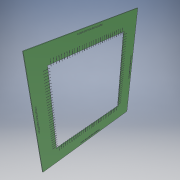
# Autodesk Inventor part: PCB-FerriteCore#01
Saved by Autodesk Inventor 2018 (Build 220112000, 112)
## iProperties
Created: 2025-02-18
Part Number: PCB-FerriteCore#01
Material: Železo, lité
Document SubType Name: Modeling
Designer: Jozko Mrkvicka
Density: 7.15 g/cm^3
Appearance: Železo – šedé
Author: Jozko Mrkvicka
Autodesk Inventor part; units mm, degrees
(part 1 of 3)
ref_plane "YZ Plane" through (0, 0, 0) normal (1, 0, 0) x (0, 1, 0)
ref_plane "XZ Plane" through (0, 0, 0) normal (0, 1, 0) x (-1, 0, 0)
ref_plane "XY Plane" through (0, 0, 0) normal (0, 0, 1) x (1, 0, 0)
sketch "Náčrt1" plane through (0, 0, 0) normal (0, 1, 0) x (-1, 0, 0)
  line L0 (-177.8, 177.8) -> (177.8, 177.8)
  line L1 (177.8, 177.8) -> (177.8, -177.8)
  line L2 (177.8, -177.8) -> (-177.8, -177.8)
  line L3 (-177.8, -177.8) -> (-177.8, 177.8)
  line L4 (-177.8, 177.8) -> (177.8, -177.8) construction
  line L5 (177.8, 177.8) -> (-177.8, -177.8) construction
  line L6 (-127, 127) -> (127, 127)
  line L7 (127, 127) -> (127, -127)
  line L8 (127, -127) -> (-127, -127)
  line L9 (-127, -127) -> (-127, 127)
  line L10 (-127, 127) -> (127, -127) construction
  line L11 (127, 127) -> (-127, -127) construction
  point P0 (0, 0)
  dimension "d2" = 355.6
  dimension "d3" = 355.6
  dimension "d4" = 254
  dimension "d5" = 254
  constraints: 24 end point, 4 midpoint, 4 parallel, 2 horizontal, 2 perpendicular
  measures "d2" distance of L1.end L2.end
  measures "d3" distance of L0.end L1.end
  measures "d4" distance of L7.end L8.end
  measures "d5" distance of L6.end L7.end
extrude "Vysunutí1" add sketch "Náčrt1" along normal blind 2.54
sketch "Náčrt2" plane through (0, 2.54, 0) normal (0, 1, 0) x (1, 0, 0)
  line L0 (88.9, -88.9) -> (-88.9, -88.9)
  line L1 (3.71, -139.7) -> (3.91, -139.7)
  line L2 (3.91, -139.7) -> (3.91, -121.92)
  line L3 (3.91, -121.92) -> (3.71, -121.92)
  line L4 (3.71, -121.92) -> (3.71, -139.7)
  line L5 (3.71, -139.7) -> (3.91, -121.92) construction
  line L6 (3.91, -139.7) -> (3.71, -121.92) construction
  line L7 (-248.92, 0) -> (248.92, 0) projected
  line L8 (0, 248.92) -> (0, -248.92) projected
  line L9 (3.71, 139.7) -> (3.91, 139.7)
  line L10 (3.91, 139.7) -> (3.91, 121.92)
  line L11 (3.91, 121.92) -> (3.71, 121.92)
  line L12 (3.71, 121.92) -> (3.71, 139.7)
  point P0 (0, 0)
  point P1 (3.81, -130.81)
  dimension "d18" = 3.81
  dimension "d19" = 0.2
  dimension "d20" = 17.78
  dimension "d24" = 139.7
  constraints: 22 end point, 4 symmetric about line, 3 parallel, 2 midpoint, 1 perpendicular
  measures "d18" horizontal distance of point (0, 0) point (3.81, -130.81)
  measures "d19" distance of L2.end L3.end
  measures "d20" distance of L1.end L2.end
  measures "d24" distance from line of L1 point (0, 0)
extrude "Vysunutí2" add sketch "Náčrt2" along normal blind 0.2
pattern_linear "Obdélníkové pole2" count 32 spacing 7.62 along (-1, 0, 0) of "Vysunutí2" first direction both ways yes
sketch "Náčrt3" plane through (0, 2.54, 0) normal (0, 1, 0) x (1, 0, 0)
  line L0 (-248.92, 0) -> (248.92, 0) projected
  line L1 (0, 248.92) -> (0, -248.92) projected
  line L2 (-121.92, -3.71) -> (-139.7, -3.71)
  line L3 (-139.7, -3.71) -> (-139.7, -3.91)
  line L4 (-139.7, -3.91) -> (-121.92, -3.91)
  line L5 (-121.92, -3.91) -> (-121.92, -3.71)
  line L6 (-121.92, -3.71) -> (-139.7, -3.91) construction
  line L7 (-139.7, -3.71) -> (-121.92, -3.91) construction
  line L8 (121.92, -3.71) -> (139.7, -3.71)
  line L9 (139.7, -3.71) -> (139.7, -3.91)
  line L10 (139.7, -3.91) -> (121.92, -3.91)
  line L11 (121.92, -3.91) -> (121.92, -3.71)
  point P0 (0, 0)
  point P1 (-130.81, -3.81)
  dimension "d35" = 0.2
  dimension "d36" = 17.78
  dimension "d37" = 3.81
  dimension "d38" = 139.7
  constraints: 20 end point, 4 symmetric about line, 2 midpoint, 2 parallel, 1 horizontal, 1 perpendicular
  measures "d35" distance of L4.end L2.start
  measures "d36" distance of L3.end L4.end
  measures "d37" distance from line of L0 point (-130.81, -3.81)
  measures "d38" distance between parallel lines of L1 L3
extrude "Vysunutí3" add sketch "Náčrt3" along normal blind 0.2
pattern_linear "Obdélníkové pole3" count 32 spacing 7.62 along (0, 0, -1) of "Vysunutí3" first direction both ways yes
sketch "Náčrt5" plane through (0, 2.54, 0) normal (0, 1, 0) x (1, 0, 0)
  line L0 (-248.92, 0) -> (248.92, 0) projected
  line L1 (172.72, -40.64) -> (167.64, -40.64)
  line L2 (167.64, -40.64) -> (167.64, 40.64)
  line L3 (167.64, 40.64) -> (172.72, 40.64)
  line L4 (172.72, 40.64) -> (172.72, -40.64)
  line L5 (172.72, -40.64) -> (167.64, 40.64) construction
  line L6 (167.64, -40.64) -> (172.72, 40.64) construction
  line L7 (177.8, -177.8) -> (177.8, 177.8) projected
  line L8 (177.8, 177.8) -> (-177.8, 177.8) projected
  line L9 (-177.8, 177.8) -> (-177.8, -177.8) projected
  line L10 (169.2275, 39.6875) -> (168.5925, 39.6875)
  line L11 (168.5925, 39.6875) -> (168.5925, 39.0525)
  line L12 (168.5925, 39.0525) -> (169.2275, 39.0525)
  line L13 (169.2275, 39.0525) -> (169.2275, 39.6875)
  line L14 (169.2275, 39.6875) -> (168.5925, 39.0525) construction
  line L15 (168.5925, 39.6875) -> (169.2275, 39.0525) construction
  line L16 (0, 248.92) -> (0, -248.92) projected
  line L17 (40.64, -167.64) -> (-40.64, -167.64)
  line L18 (-40.64, -167.64) -> (-40.64, -172.72)
  line L19 (-40.64, -172.72) -> (40.64, -172.72)
  line L20 (40.64, -172.72) -> (40.64, -167.64)
  line L21 (40.64, -167.64) -> (-40.64, -172.72) construction
  line L22 (-40.64, -167.64) -> (40.64, -172.72) construction
  line L23 (-177.8, -177.8) -> (177.8, -177.8) projected
  line L24 (40.64, 172.72) -> (-40.64, 172.72)
  line L25 (-40.64, 172.72) -> (-40.64, 167.64)
  line L26 (-40.64, 167.64) -> (40.64, 167.64)
  line L27 (40.64, 167.64) -> (40.64, 172.72)
  line L28 (40.64, 172.72) -> (-40.64, 167.64) construction
  line L29 (-40.64, 172.72) -> (40.64, 167.64) construction
  line L30 (-39.0525, -171.1325) -> (-39.6875, -171.1325)
  line L31 (-39.6875, -171.1325) -> (-39.6875, -171.7675)
  line L32 (-39.6875, -171.7675) -> (-39.0525, -171.7675)
  line L33 (-39.0525, -171.7675) -> (-39.0525, -171.1325)
  line L34 (-39.0525, -171.1325) -> (-39.6875, -171.7675) construction
  line L35 (-39.6875, -171.1325) -> (-39.0525, -171.7675) construction
  line L36 (-36.5125, -171.1325) -> (-37.1475, -171.1325)
  line L37 (-36.5125, -171.7675) -> (-36.5125, -171.1325)
  line L38 (-37.1475, -171.1325) -> (-37.1475, -171.7675)
  line L39 (-37.1475, -171.7675) -> (-36.5125, -171.7675)
  line L40 (-36.5125, -171.1325) -> (-37.1475, -171.7675) construction
  line L41 (-37.1475, -171.1325) -> (-36.5125, -171.7675) construction
  line L42 (-33.9725, -171.1325) -> (-34.6075, -171.1325)
  line L43 (-33.9725, -171.7675) -> (-33.9725, -171.1325)
  line L44 (-34.6075, -171.1325) -> (-34.6075, -171.7675)
  line L45 (-34.6075, -171.7675) -> (-33.9725, -171.7675)
  line L46 (-33.9725, -171.1325) -> (-34.6075, -171.7675) construction
  line L47 (-34.6075, -171.1325) -> (-33.9725, -171.7675) construction
  line L48 (-31.4325, -171.1325) -> (-32.0675, -171.1325)
  line L49 (-31.4325, -171.7675) -> (-31.4325, -171.1325)
  line L50 (-32.0675, -171.1325) -> (-32.0675, -171.7675)
  line L51 (-32.0675, -171.7675) -> (-31.4325, -171.7675)
  line L52 (-31.4325, -171.1325) -> (-32.0675, -171.7675) construction
  line L53 (-32.0675, -171.1325) -> (-31.4325, -171.7675) construction
  line L54 (-28.8925, -171.1325) -> (-29.5275, -171.1325)
  line L55 (-28.8925, -171.7675) -> (-28.8925, -171.1325)
  line L56 (-29.5275, -171.1325) -> (-29.5275, -171.7675)
  line L57 (-29.5275, -171.7675) -> (-28.8925, -171.7675)
  line L58 (-28.8925, -171.1325) -> (-29.5275, -171.7675) construction
  line L59 (-29.5275, -171.1325) -> (-28.8925, -171.7675) construction
  line L60 (-26.3525, -171.1325) -> (-26.9875, -171.1325)
  line L61 (-26.3525, -171.7675) -> (-26.3525, -171.1325)
  line L62 (-26.9875, -171.1325) -> (-26.9875, -171.7675)
  line L63 (-26.9875, -171.7675) -> (-26.3525, -171.7675)
  line L64 (-26.3525, -171.1325) -> (-26.9875, -171.7675) construction
  line L65 (-26.9875, -171.1325) -> (-26.3525, -171.7675) construction
  line L66 (-23.8125, -171.1325) -> (-24.4475, -171.1325)
  line L67 (-23.8125, -171.7675) -> (-23.8125, -171.1325)
  line L68 (-24.4475, -171.1325) -> (-24.4475, -171.7675)
  line L69 (-24.4475, -171.7675) -> (-23.8125, -171.7675)
  line L70 (-23.8125, -171.1325) -> (-24.4475, -171.7675) construction
  line L71 (-24.4475, -171.1325) -> (-23.8125, -171.7675) construction
  line L72 (-21.2725, -171.1325) -> (-21.9075, -171.1325)
  line L73 (-21.2725, -171.7675) -> (-21.2725, -171.1325)
  line L74 (-21.9075, -171.1325) -> (-21.9075, -171.7675)
  line L75 (-21.9075, -171.7675) -> (-21.2725, -171.7675)
  line L76 (-21.2725, -171.1325) -> (-21.9075, -171.7675) construction
  line L77 (-21.9075, -171.1325) -> (-21.2725, -171.7675) construction
  line L78 (-18.7325, -171.1325) -> (-19.3675, -171.1325)
  line L79 (-18.7325, -171.7675) -> (-18.7325, -171.1325)
  line L80 (-19.3675, -171.1325) -> (-19.3675, -171.7675)
  line L81 (-19.3675, -171.7675) -> (-18.7325, -171.7675)
  line L82 (-18.7325, -171.1325) -> (-19.3675, -171.7675) construction
  line L83 (-19.3675, -171.1325) -> (-18.7325, -171.7675) construction
  line L84 (-16.1925, -171.1325) -> (-16.8275, -171.1325)
  line L85 (-16.1925, -171.7675) -> (-16.1925, -171.1325)
  line L86 (-16.8275, -171.1325) -> (-16.8275, -171.7675)
  line L87 (-16.8275, -171.7675) -> (-16.1925, -171.7675)
  line L88 (-16.1925, -171.1325) -> (-16.8275, -171.7675) construction
  line L89 (-16.8275, -171.1325) -> (-16.1925, -171.7675) construction
  line L90 (-13.6525, -171.1325) -> (-14.2875, -171.1325)
  line L91 (-13.6525, -171.7675) -> (-13.6525, -171.1325)
  line L92 (-14.2875, -171.1325) -> (-14.2875, -171.7675)
  line L93 (-14.2875, -171.7675) -> (-13.6525, -171.7675)
  line L94 (-13.6525, -171.1325) -> (-14.2875, -171.7675) construction
  line L95 (-14.2875, -171.1325) -> (-13.6525, -171.7675) construction
  line L96 (-11.1125, -171.1325) -> (-11.7475, -171.1325)
  line L97 (-11.1125, -171.7675) -> (-11.1125, -171.1325)
  line L98 (-11.7475, -171.1325) -> (-11.7475, -171.7675)
  line L99 (-11.7475, -171.7675) -> (-11.1125, -171.7675)
  line L100 (-11.1125, -171.1325) -> (-11.7475, -171.7675) construction
  line L101 (-11.7475, -171.1325) -> (-11.1125, -171.7675) construction
  line L102 (-8.5725, -171.1325) -> (-9.2075, -171.1325)
  line L103 (-8.5725, -171.7675) -> (-8.5725, -171.1325)
  line L104 (-9.2075, -171.1325) -> (-9.2075, -171.7675)
  line L105 (-9.2075, -171.7675) -> (-8.5725, -171.7675)
  line L106 (-8.5725, -171.1325) -> (-9.2075, -171.7675) construction
  line L107 (-9.2075, -171.1325) -> (-8.5725, -171.7675) construction
  line L108 (-6.0325, -171.1325) -> (-6.6675, -171.1325)
  line L109 (-6.0325, -171.7675) -> (-6.0325, -171.1325)
  line L110 (-6.6675, -171.1325) -> (-6.6675, -171.7675)
  line L111 (-6.6675, -171.7675) -> (-6.0325, -171.7675)
  line L112 (-6.0325, -171.1325) -> (-6.6675, -171.7675) construction
  line L113 (-6.6675, -171.1325) -> (-6.0325, -171.7675) construction
  line L114 (-3.4925, -171.1325) -> (-4.1275, -171.1325)
  line L115 (-3.4925, -171.7675) -> (-3.4925, -171.1325)
  line L116 (-4.1275, -171.1325) -> (-4.1275, -171.7675)
  line L117 (-4.1275, -171.7675) -> (-3.4925, -171.7675)
  line L118 (-3.4925, -171.1325) -> (-4.1275, -171.7675) construction
  line L119 (-4.1275, -171.1325) -> (-3.4925, -171.7675) construction
  line L120 (-0.9525, -171.1325) -> (-1.5875, -171.1325)
  line L121 (-0.9525, -171.7675) -> (-0.9525, -171.1325)
  line L122 (-1.5875, -171.1325) -> (-1.5875, -171.7675)
  line L123 (-1.5875, -171.7675) -> (-0.9525, -171.7675)
  line L124 (-0.9525, -171.1325) -> (-1.5875, -171.7675) construction
  line L125 (-1.5875, -171.1325) -> (-0.9525, -171.7675) construction
  line L126 (1.5875, -171.1325) -> (0.9525, -171.1325)
  line L127 (1.5875, -171.7675) -> (1.5875, -171.1325)
  line L128 (0.9525, -171.1325) -> (0.9525, -171.7675)
  line L129 (0.9525, -171.7675) -> (1.5875, -171.7675)
  line L130 (1.5875, -171.1325) -> (0.9525, -171.7675) construction
  line L131 (0.9525, -171.1325) -> (1.5875, -171.7675) construction
  line L132 (4.1275, -171.1325) -> (3.4925, -171.1325)
  line L133 (4.1275, -171.7675) -> (4.1275, -171.1325)
  line L134 (3.4925, -171.1325) -> (3.4925, -171.7675)
  line L135 (3.4925, -171.7675) -> (4.1275, -171.7675)
  line L136 (4.1275, -171.1325) -> (3.4925, -171.7675) construction
  line L137 (3.4925, -171.1325) -> (4.1275, -171.7675) construction
  line L138 (6.6675, -171.1325) -> (6.0325, -171.1325)
  line L139 (6.6675, -171.7675) -> (6.6675, -171.1325)
  line L140 (6.0325, -171.1325) -> (6.0325, -171.7675)
  line L141 (6.0325, -171.7675) -> (6.6675, -171.7675)
  line L142 (6.6675, -171.1325) -> (6.0325, -171.7675) construction
  line L143 (6.0325, -171.1325) -> (6.6675, -171.7675) construction
  line L144 (9.2075, -171.1325) -> (8.5725, -171.1325)
  line L145 (9.2075, -171.7675) -> (9.2075, -171.1325)
  line L146 (8.5725, -171.1325) -> (8.5725, -171.7675)
  line L147 (8.5725, -171.7675) -> (9.2075, -171.7675)
  line L148 (9.2075, -171.1325) -> (8.5725, -171.7675) construction
  line L149 (8.5725, -171.1325) -> (9.2075, -171.7675) construction
  line L150 (11.7475, -171.1325) -> (11.1125, -171.1325)
  line L151 (11.7475, -171.7675) -> (11.7475, -171.1325)
  line L152 (11.1125, -171.1325) -> (11.1125, -171.7675)
  line L153 (11.1125, -171.7675) -> (11.7475, -171.7675)
  line L154 (11.7475, -171.1325) -> (11.1125, -171.7675) construction
  line L155 (11.1125, -171.1325) -> (11.7475, -171.7675) construction
  line L156 (14.2875, -171.1325) -> (13.6525, -171.1325)
  line L157 (14.2875, -171.7675) -> (14.2875, -171.1325)
  line L158 (13.6525, -171.1325) -> (13.6525, -171.7675)
  line L159 (13.6525, -171.7675) -> (14.2875, -171.7675)
  line L160 (14.2875, -171.1325) -> (13.6525, -171.7675) construction
  line L161 (13.6525, -171.1325) -> (14.2875, -171.7675) construction
  line L162 (16.8275, -171.1325) -> (16.1925, -171.1325)
  line L163 (16.8275, -171.7675) -> (16.8275, -171.1325)
  line L164 (16.1925, -171.1325) -> (16.1925, -171.7675)
  line L165 (16.1925, -171.7675) -> (16.8275, -171.7675)
  line L166 (16.8275, -171.1325) -> (16.1925, -171.7675) construction
  line L167 (16.1925, -171.1325) -> (16.8275, -171.7675) construction
  line L168 (19.3675, -171.1325) -> (18.7325, -171.1325)
  line L169 (19.3675, -171.7675) -> (19.3675, -171.1325)
  line L170 (18.7325, -171.1325) -> (18.7325, -171.7675)
  line L171 (18.7325, -171.7675) -> (19.3675, -171.7675)
  line L172 (19.3675, -171.1325) -> (18.7325, -171.7675) construction
  line L173 (18.7325, -171.1325) -> (19.3675, -171.7675) construction
  line L174 (21.9075, -171.1325) -> (21.2725, -171.1325)
  line L175 (21.9075, -171.7675) -> (21.9075, -171.1325)
  line L176 (21.2725, -171.1325) -> (21.2725, -171.7675)
  line L177 (21.2725, -171.7675) -> (21.9075, -171.7675)
  line L178 (21.9075, -171.1325) -> (21.2725, -171.7675) construction
  line L179 (21.2725, -171.1325) -> (21.9075, -171.7675) construction
  line L180 (24.4475, -171.1325) -> (23.8125, -171.1325)
  line L181 (24.4475, -171.7675) -> (24.4475, -171.1325)
  line L182 (23.8125, -171.1325) -> (23.8125, -171.7675)
  line L183 (23.8125, -171.7675) -> (24.4475, -171.7675)
  line L184 (24.4475, -171.1325) -> (23.8125, -171.7675) construction
  line L185 (23.8125, -171.1325) -> (24.4475, -171.7675) construction
  line L186 (26.9875, -171.1325) -> (26.3525, -171.1325)
  line L187 (26.9875, -171.7675) -> (26.9875, -171.1325)
  line L188 (26.3525, -171.1325) -> (26.3525, -171.7675)
  line L189 (26.3525, -171.7675) -> (26.9875, -171.7675)
  line L190 (26.9875, -171.1325) -> (26.3525, -171.7675) construction
  line L191 (26.3525, -171.1325) -> (26.9875, -171.7675) construction
  line L192 (29.5275, -171.1325) -> (28.8925, -171.1325)
  line L193 (29.5275, -171.7675) -> (29.5275, -171.1325)
  line L194 (28.8925, -171.1325) -> (28.8925, -171.7675)
  line L195 (28.8925, -171.7675) -> (29.5275, -171.7675)
  line L196 (29.5275, -171.1325) -> (28.8925, -171.7675) construction
  line L197 (28.8925, -171.1325) -> (29.5275, -171.7675) construction
  line L198 (32.0675, -171.1325) -> (31.4325, -171.1325)
  line L199 (32.0675, -171.7675) -> (32.0675, -171.1325)
  line L200 (31.4325, -171.1325) -> (31.4325, -171.7675)
  line L201 (31.4325, -171.7675) -> (32.0675, -171.7675)
  line L202 (32.0675, -171.1325) -> (31.4325, -171.7675) construction
  line L203 (31.4325, -171.1325) -> (32.0675, -171.7675) construction
  line L204 (34.6075, -171.1325) -> (33.9725, -171.1325)
  line L205 (34.6075, -171.7675) -> (34.6075, -171.1325)
  line L206 (33.9725, -171.1325) -> (33.9725, -171.7675)
  line L207 (33.9725, -171.7675) -> (34.6075, -171.7675)
  line L208 (34.6075, -171.1325) -> (33.9725, -171.7675) construction
  line L209 (33.9725, -171.1325) -> (34.6075, -171.7675) construction
  line L210 (37.1475, -171.1325) -> (36.5125, -171.1325)
  line L211 (37.1475, -171.7675) -> (37.1475, -171.1325)
  line L212 (36.5125, -171.1325) -> (36.5125, -171.7675)
  line L213 (36.5125, -171.7675) -> (37.1475, -171.7675)
  line L214 (37.1475, -171.1325) -> (36.5125, -171.7675) construction
  line L215 (36.5125, -171.1325) -> (37.1475, -171.7675) construction
  line L216 (39.6875, -171.1325) -> (39.0525, -171.1325)
  line L217 (39.6875, -171.7675) -> (39.6875, -171.1325)
  line L218 (39.0525, -171.1325) -> (39.0525, -171.7675)
  line L219 (39.0525, -171.7675) -> (39.6875, -171.7675)
  line L220 (39.6875, -171.1325) -> (39.0525, -171.7675) construction
  line L221 (39.0525, -171.1325) -> (39.6875, -171.7675) construction
  line L222 (-39.0525, -168.5925) -> (-39.6875, -168.5925)
  line L223 (-39.0525, -169.2275) -> (-39.0525, -168.5925)
  line L224 (-39.6875, -168.5925) -> (-39.6875, -169.2275)
  line L225 (-39.6875, -169.2275) -> (-39.0525, -169.2275)
  line L226 (-39.0525, -168.5925) -> (-39.6875, -169.2275) construction
  line L227 (-39.6875, -168.5925) -> (-39.0525, -169.2275) construction
  line L228 (-36.5125, -168.5925) -> (-37.1475, -168.5925)
  line L229 (-36.5125, -169.2275) -> (-36.5125, -168.5925)
  line L230 (-37.1475, -168.5925) -> (-37.1475, -169.2275)
  line L231 (-37.1475, -169.2275) -> (-36.5125, -169.2275)
  line L232 (-36.5125, -168.5925) -> (-37.1475, -169.2275) construction
  line L233 (-37.1475, -168.5925) -> (-36.5125, -169.2275) construction
  line L234 (-33.9725, -168.5925) -> (-34.6075, -168.5925)
  line L235 (-33.9725, -169.2275) -> (-33.9725, -168.5925)
  line L236 (-34.6075, -168.5925) -> (-34.6075, -169.2275)
  line L237 (-34.6075, -169.2275) -> (-33.9725, -169.2275)
  line L238 (-33.9725, -168.5925) -> (-34.6075, -169.2275) construction
  line L239 (-34.6075, -168.5925) -> (-33.9725, -169.2275) construction
  line L240 (-31.4325, -168.5925) -> (-32.0675, -168.5925)
  line L241 (-31.4325, -169.2275) -> (-31.4325, -168.5925)
  line L242 (-32.0675, -168.5925) -> (-32.0675, -169.2275)
  line L243 (-32.0675, -169.2275) -> (-31.4325, -169.2275)
  line L244 (-31.4325, -168.5925) -> (-32.0675, -169.2275) construction
  line L245 (-32.0675, -168.5925) -> (-31.4325, -169.2275) construction
  line L246 (-28.8925, -168.5925) -> (-29.5275, -168.5925)
  line L247 (-28.8925, -169.2275) -> (-28.8925, -168.5925)
  line L248 (-29.5275, -168.5925) -> (-29.5275, -169.2275)
  line L249 (-29.5275, -169.2275) -> (-28.8925, -169.2275)
  line L250 (-28.8925, -168.5925) -> (-29.5275, -169.2275) construction
  line L251 (-29.5275, -168.5925) -> (-28.8925, -169.2275) construction
  line L252 (-26.3525, -168.5925) -> (-26.9875, -168.5925)
  line L253 (-26.3525, -169.2275) -> (-26.3525, -168.5925)
  line L254 (-26.9875, -168.5925) -> (-26.9875, -169.2275)
  line L255 (-26.9875, -169.2275) -> (-26.3525, -169.2275)
  line L256 (-26.3525, -168.5925) -> (-26.9875, -169.2275) construction
  line L257 (-26.9875, -168.5925) -> (-26.3525, -169.2275) construction
  line L258 (-23.8125, -168.5925) -> (-24.4475, -168.5925)
  line L259 (-23.8125, -169.2275) -> (-23.8125, -168.5925)
  line L260 (-24.4475, -168.5925) -> (-24.4475, -169.2275)
  line L261 (-24.4475, -169.2275) -> (-23.8125, -169.2275)
  line L262 (-23.8125, -168.5925) -> (-24.4475, -169.2275) construction
  line L263 (-24.4475, -168.5925) -> (-23.8125, -169.2275) construction
  line L264 (-21.2725, -168.5925) -> (-21.9075, -168.5925)
  line L265 (-21.2725, -169.2275) -> (-21.2725, -168.5925)
  line L266 (-21.9075, -168.5925) -> (-21.9075, -169.2275)
  line L267 (-21.9075, -169.2275) -> (-21.2725, -169.2275)
  line L268 (-21.2725, -168.5925) -> (-21.9075, -169.2275) construction
  line L269 (-21.9075, -168.5925) -> (-21.2725, -169.2275) construction
  line L270 (-18.7325, -168.5925) -> (-19.3675, -168.5925)
  line L271 (-18.7325, -169.2275) -> (-18.7325, -168.5925)
  line L272 (-19.3675, -168.5925) -> (-19.3675, -169.2275)
  line L273 (-19.3675, -169.2275) -> (-18.7325, -169.2275)
  line L274 (-18.7325, -168.5925) -> (-19.3675, -169.2275) construction
  line L275 (-19.3675, -168.5925) -> (-18.7325, -169.2275) construction
  line L276 (-16.1925, -168.5925) -> (-16.8275, -168.5925)
  line L277 (-16.1925, -169.2275) -> (-16.1925, -168.5925)
  line L278 (-16.8275, -168.5925) -> (-16.8275, -169.2275)
  line L279 (-16.8275, -169.2275) -> (-16.1925, -169.2275)
  line L280 (-16.1925, -168.5925) -> (-16.8275, -169.2275) construction
  line L281 (-16.8275, -168.5925) -> (-16.1925, -169.2275) construction
  line L282 (-13.6525, -168.5925) -> (-14.2875, -168.5925)
  line L283 (-13.6525, -169.2275) -> (-13.6525, -168.5925)
  line L284 (-14.2875, -168.5925) -> (-14.2875, -169.2275)
  line L285 (-14.2875, -169.2275) -> (-13.6525, -169.2275)
  line L286 (-13.6525, -168.5925) -> (-14.2875, -169.2275) construction
  line L287 (-14.2875, -168.5925) -> (-13.6525, -169.2275) construction
  line L288 (-11.1125, -168.5925) -> (-11.7475, -168.5925)
  line L289 (-11.1125, -169.2275) -> (-11.1125, -168.5925)
  line L290 (-11.7475, -168.5925) -> (-11.7475, -169.2275)
  line L291 (-11.7475, -169.2275) -> (-11.1125, -169.2275)
  line L292 (-11.1125, -168.5925) -> (-11.7475, -169.2275) construction
  line L293 (-11.7475, -168.5925) -> (-11.1125, -169.2275) construction
  line L294 (-8.5725, -168.5925) -> (-9.2075, -168.5925)
  line L295 (-8.5725, -169.2275) -> (-8.5725, -168.5925)
  line L296 (-9.2075, -168.5925) -> (-9.2075, -169.2275)
  line L297 (-9.2075, -169.2275) -> (-8.5725, -169.2275)
  line L298 (-8.5725, -168.5925) -> (-9.2075, -169.2275) construction
  line L299 (-9.2075, -168.5925) -> (-8.5725, -169.2275) construction
  line L300 (-6.0325, -168.5925) -> (-6.6675, -168.5925)
  line L301 (-6.0325, -169.2275) -> (-6.0325, -168.5925)
  line L302 (-6.6675, -168.5925) -> (-6.6675, -169.2275)
  line L303 (-6.6675, -169.2275) -> (-6.0325, -169.2275)
  line L304 (-6.0325, -168.5925) -> (-6.6675, -169.2275) construction
  line L305 (-6.6675, -168.5925) -> (-6.0325, -169.2275) construction
  line L306 (-3.4925, -168.5925) -> (-4.1275, -168.5925)
  line L307 (-3.4925, -169.2275) -> (-3.4925, -168.5925)
  line L308 (-4.1275, -168.5925) -> (-4.1275, -169.2275)
  line L309 (-4.1275, -169.2275) -> (-3.4925, -169.2275)
  line L310 (-3.4925, -168.5925) -> (-4.1275, -169.2275) construction
  line L311 (-4.1275, -168.5925) -> (-3.4925, -169.2275) construction
  line L312 (-0.9525, -168.5925) -> (-1.5875, -168.5925)
  line L313 (-0.9525, -169.2275) -> (-0.9525, -168.5925)
  line L314 (-1.5875, -168.5925) -> (-1.5875, -169.2275)
  line L315 (-1.5875, -169.2275) -> (-0.9525, -169.2275)
  line L316 (-0.9525, -168.5925) -> (-1.5875, -169.2275) construction
  line L317 (-1.5875, -168.5925) -> (-0.9525, -169.2275) construction
  line L318 (1.5875, -168.5925) -> (0.9525, -168.5925)
  line L319 (1.5875, -169.2275) -> (1.5875, -168.5925)
  line L320 (0.9525, -168.5925) -> (0.9525, -169.2275)
  line L321 (0.9525, -169.2275) -> (1.5875, -169.2275)
  line L322 (1.5875, -168.5925) -> (0.9525, -169.2275) construction
  line L323 (0.9525, -168.5925) -> (1.5875, -169.2275) construction
  line L324 (4.1275, -168.5925) -> (3.4925, -168.5925)
  line L325 (4.1275, -169.2275) -> (4.1275, -168.5925)
  line L326 (3.4925, -168.5925) -> (3.4925, -169.2275)
  line L327 (3.4925, -169.2275) -> (4.1275, -169.2275)
  line L328 (4.1275, -168.5925) -> (3.4925, -169.2275) construction
  line L329 (3.4925, -168.5925) -> (4.1275, -169.2275) construction
  line L330 (6.6675, -168.5925) -> (6.0325, -168.5925)
  line L331 (6.6675, -169.2275) -> (6.6675, -168.5925)
  line L332 (6.0325, -168.5925) -> (6.0325, -169.2275)
  line L333 (6.0325, -169.2275) -> (6.6675, -169.2275)
  line L334 (6.6675, -168.5925) -> (6.0325, -169.2275) construction
  line L335 (6.0325, -168.5925) -> (6.6675, -169.2275) construction
  line L336 (9.2075, -168.5925) -> (8.5725, -168.5925)
  line L337 (9.2075, -169.2275) -> (9.2075, -168.5925)
  line L338 (8.5725, -168.5925) -> (8.5725, -169.2275)
  line L339 (8.5725, -169.2275) -> (9.2075, -169.2275)
  line L340 (9.2075, -168.5925) -> (8.5725, -169.2275) construction
  line L341 (8.5725, -168.5925) -> (9.2075, -169.2275) construction
  line L342 (11.7475, -168.5925) -> (11.1125, -168.5925)
  line L343 (11.7475, -169.2275) -> (11.7475, -168.5925)
  line L344 (11.1125, -168.5925) -> (11.1125, -169.2275)
  line L345 (11.1125, -169.2275) -> (11.7475, -169.2275)
  line L346 (11.7475, -168.5925) -> (11.1125, -169.2275) construction
  line L347 (11.1125, -168.5925) -> (11.7475, -169.2275) construction
  line L348 (14.2875, -168.5925) -> (13.6525, -168.5925)
  line L349 (14.2875, -169.2275) -> (14.2875, -168.5925)
  line L350 (13.6525, -168.5925) -> (13.6525, -169.2275)
  line L351 (13.6525, -169.2275) -> (14.2875, -169.2275)
  line L352 (14.2875, -168.5925) -> (13.6525, -169.2275) construction
  line L353 (13.6525, -168.5925) -> (14.2875, -169.2275) construction
  line L354 (16.8275, -168.5925) -> (16.1925, -168.5925)
  line L355 (16.8275, -169.2275) -> (16.8275, -168.5925)
  line L356 (16.1925, -168.5925) -> (16.1925, -169.2275)
  line L357 (16.1925, -169.2275) -> (16.8275, -169.2275)
  line L358 (16.8275, -168.5925) -> (16.1925, -169.2275) construction
  line L359 (16.1925, -168.5925) -> (16.8275, -169.2275) construction
  line L360 (19.3675, -168.5925) -> (18.7325, -168.5925)
  line L361 (19.3675, -169.2275) -> (19.3675, -168.5925)
  line L362 (18.7325, -168.5925) -> (18.7325, -169.2275)
  line L363 (18.7325, -169.2275) -> (19.3675, -169.2275)
  line L364 (19.3675, -168.5925) -> (18.7325, -169.2275) construction
  line L365 (18.7325, -168.5925) -> (19.3675, -169.2275) construction
  line L366 (21.9075, -168.5925) -> (21.2725, -168.5925)
  line L367 (21.9075, -169.2275) -> (21.9075, -168.5925)
  line L368 (21.2725, -168.5925) -> (21.2725, -169.2275)
  line L369 (21.2725, -169.2275) -> (21.9075, -169.2275)
  line L370 (21.9075, -168.5925) -> (21.2725, -169.2275) construction
  line L371 (21.2725, -168.5925) -> (21.9075, -169.2275) construction
  line L372 (24.4475, -168.5925) -> (23.8125, -168.5925)
  line L373 (24.4475, -169.2275) -> (24.4475, -168.5925)
  line L374 (23.8125, -168.5925) -> (23.8125, -169.2275)
  line L375 (23.8125, -169.2275) -> (24.4475, -169.2275)
  line L376 (24.4475, -168.5925) -> (23.8125, -169.2275) construction
  line L377 (23.8125, -168.5925) -> (24.4475, -169.2275) construction
  line L378 (26.9875, -168.5925) -> (26.3525, -168.5925)
  line L379 (26.9875, -169.2275) -> (26.9875, -168.5925)
  line L380 (26.3525, -168.5925) -> (26.3525, -169.2275)
  line L381 (26.3525, -169.2275) -> (26.9875, -169.2275)
  line L382 (26.9875, -168.5925) -> (26.3525, -169.2275) construction
  line L383 (26.3525, -168.5925) -> (26.9875, -169.2275) construction
  line L384 (29.5275, -168.5925) -> (28.8925, -168.5925)
  line L385 (29.5275, -169.2275) -> (29.5275, -168.5925)
  line L386 (28.8925, -168.5925) -> (28.8925, -169.2275)
  line L387 (28.8925, -169.2275) -> (29.5275, -169.2275)
  line L388 (29.5275, -168.5925) -> (28.8925, -169.2275) construction
  line L389 (28.8925, -168.5925) -> (29.5275, -169.2275) construction
  line L390 (32.0675, -168.5925) -> (31.4325, -168.5925)
  line L391 (32.0675, -169.2275) -> (32.0675, -168.5925)
  line L392 (31.4325, -168.5925) -> (31.4325, -169.2275)
  line L393 (31.4325, -169.2275) -> (32.0675, -169.2275)
  line L394 (32.0675, -168.5925) -> (31.4325, -169.2275) construction
  line L395 (31.4325, -168.5925) -> (32.0675, -169.2275) construction
  line L396 (34.6075, -168.5925) -> (33.9725, -168.5925)
  line L397 (34.6075, -169.2275) -> (34.6075, -168.5925)
  line L398 (33.9725, -168.5925) -> (33.9725, -169.2275)
  line L399 (33.9725, -169.2275) -> (34.6075, -169.2275)
  line L400 (34.6075, -168.5925) -> (33.9725, -169.2275) construction
  line L401 (33.9725, -168.5925) -> (34.6075, -169.2275) construction
  line L402 (37.1475, -168.5925) -> (36.5125, -168.5925)
  line L403 (37.1475, -169.2275) -> (37.1475, -168.5925)
  line L404 (36.5125, -168.5925) -> (36.5125, -169.2275)
  line L405 (36.5125, -169.2275) -> (37.1475, -169.2275)
  line L406 (37.1475, -168.5925) -> (36.5125, -169.2275) construction
  line L407 (36.5125, -168.5925) -> (37.1475, -169.2275) construction
  line L408 (39.6875, -168.5925) -> (39.0525, -168.5925)
  line L409 (39.6875, -169.2275) -> (39.6875, -168.5925)
  line L410 (39.0525, -168.5925) -> (39.0525, -169.2275)
  line L411 (39.0525, -169.2275) -> (39.6875, -169.2275)
  line L412 (39.6875, -168.5925) -> (39.0525, -169.2275) construction
  line L413 (39.0525, -168.5925) -> (39.6875, -169.2275) construction
  line L414 (-39.0525, 169.2275) -> (-39.6875, 169.2275)
  line L415 (-39.6875, 169.2275) -> (-39.6875, 168.5925)
  line L416 (-39.6875, 168.5925) -> (-39.0525, 168.5925)
  line L417 (-39.0525, 168.5925) -> (-39.0525, 169.2275)
  line L418 (-39.0525, 169.2275) -> (-39.6875, 168.5925) construction
  line L419 (-39.6875, 169.2275) -> (-39.0525, 168.5925) construction
  line L420 (-37.1475, 168.5925) -> (-36.5125, 168.5925)
  line L421 (-36.5125, 168.5925) -> (-36.5125, 169.2275)
  line L422 (-37.1475, 169.2275) -> (-37.1475, 168.5925)
  line L423 (-36.5125, 169.2275) -> (-37.1475, 169.2275)
  line L424 (-36.5125, 169.2275) -> (-37.1475, 168.5925) construction
  line L425 (-37.1475, 169.2275) -> (-36.5125, 168.5925) construction
  line L426 (-34.6075, 168.5925) -> (-33.9725, 168.5925)
  line L427 (-33.9725, 168.5925) -> (-33.9725, 169.2275)
  line L428 (-34.6075, 169.2275) -> (-34.6075, 168.5925)
  line L429 (-33.9725, 169.2275) -> (-34.6075, 169.2275)
  line L430 (-33.9725, 169.2275) -> (-34.6075, 168.5925) construction
  line L431 (-34.6075, 169.2275) -> (-33.9725, 168.5925) construction
  line L432 (-32.0675, 168.5925) -> (-31.4325, 168.5925)
  line L433 (-31.4325, 168.5925) -> (-31.4325, 169.2275)
  line L434 (-32.0675, 169.2275) -> (-32.0675, 168.5925)
  line L435 (-31.4325, 169.2275) -> (-32.0675, 169.2275)
  line L436 (-31.4325, 169.2275) -> (-32.0675, 168.5925) construction
  line L437 (-32.0675, 169.2275) -> (-31.4325, 168.5925) construction
  line L438 (-29.5275, 168.5925) -> (-28.8925, 168.5925)
  line L439 (-28.8925, 168.5925) -> (-28.8925, 169.2275)
  line L440 (-29.5275, 169.2275) -> (-29.5275, 168.5925)
  line L441 (-28.8925, 169.2275) -> (-29.5275, 169.2275)
  line L442 (-28.8925, 169.2275) -> (-29.5275, 168.5925) construction
  line L443 (-29.5275, 169.2275) -> (-28.8925, 168.5925) construction
  line L444 (-26.9875, 168.5925) -> (-26.3525, 168.5925)
  line L445 (-26.3525, 168.5925) -> (-26.3525, 169.2275)
  line L446 (-26.9875, 169.2275) -> (-26.9875, 168.5925)
  line L447 (-26.3525, 169.2275) -> (-26.9875, 169.2275)
  line L448 (-26.3525, 169.2275) -> (-26.9875, 168.5925) construction
  line L449 (-26.9875, 169.2275) -> (-26.3525, 168.5925) construction
  line L450 (-24.4475, 168.5925) -> (-23.8125, 168.5925)
  line L451 (-23.8125, 168.5925) -> (-23.8125, 169.2275)
  line L452 (-24.4475, 169.2275) -> (-24.4475, 168.5925)
  line L453 (-23.8125, 169.2275) -> (-24.4475, 169.2275)
  line L454 (-23.8125, 169.2275) -> (-24.4475, 168.5925) construction
  line L455 (-24.4475, 169.2275) -> (-23.8125, 168.5925) construction
  line L456 (-21.9075, 168.5925) -> (-21.2725, 168.5925)
  line L457 (-21.2725, 168.5925) -> (-21.2725, 169.2275)
  line L458 (-21.9075, 169.2275) -> (-21.9075, 168.5925)
  line L459 (-21.2725, 169.2275) -> (-21.9075, 169.2275)
  line L460 (-21.2725, 169.2275) -> (-21.9075, 168.5925) construction
  line L461 (-21.9075, 169.2275) -> (-21.2725, 168.5925) construction
  line L462 (-19.3675, 168.5925) -> (-18.7325, 168.5925)
  line L463 (-18.7325, 168.5925) -> (-18.7325, 169.2275)
  line L464 (-19.3675, 169.2275) -> (-19.3675, 168.5925)
  line L465 (-18.7325, 169.2275) -> (-19.3675, 169.2275)
  line L466 (-18.7325, 169.2275) -> (-19.3675, 168.5925) construction
  line L467 (-19.3675, 169.2275) -> (-18.7325, 168.5925) construction
  line L468 (-16.8275, 168.5925) -> (-16.1925, 168.5925)
  line L469 (-16.1925, 168.5925) -> (-16.1925, 169.2275)
  line L470 (-16.8275, 169.2275) -> (-16.8275, 168.5925)
  line L471 (-16.1925, 169.2275) -> (-16.8275, 169.2275)
  line L472 (-16.1925, 169.2275) -> (-16.8275, 168.5925) construction
  line L473 (-16.8275, 169.2275) -> (-16.1925, 168.5925) construction
  line L474 (-14.2875, 168.5925) -> (-13.6525, 168.5925)
  line L475 (-13.6525, 168.5925) -> (-13.6525, 169.2275)
  line L476 (-14.2875, 169.2275) -> (-14.2875, 168.5925)
  line L477 (-13.6525, 169.2275) -> (-14.2875, 169.2275)
  line L478 (-13.6525, 169.2275) -> (-14.2875, 168.5925) construction
  line L479 (-14.2875, 169.2275) -> (-13.6525, 168.5925) construction
  line L480 (-11.7475, 168.5925) -> (-11.1125, 168.5925)
  line L481 (-11.1125, 168.5925) -> (-11.1125, 169.2275)
  line L482 (-11.7475, 169.2275) -> (-11.7475, 168.5925)
  line L483 (-11.1125, 169.2275) -> (-11.7475, 169.2275)
  line L484 (-11.1125, 169.2275) -> (-11.7475, 168.5925) construction
  line L485 (-11.7475, 169.2275) -> (-11.1125, 168.5925) construction
  line L486 (-9.2075, 168.5925) -> (-8.5725, 168.5925)
  line L487 (-8.5725, 168.5925) -> (-8.5725, 169.2275)
  line L488 (-9.2075, 169.2275) -> (-9.2075, 168.5925)
  line L489 (-8.5725, 169.2275) -> (-9.2075, 169.2275)
  line L490 (-8.5725, 169.2275) -> (-9.2075, 168.5925) construction
  line L491 (-9.2075, 169.2275) -> (-8.5725, 168.5925) construction
  line L492 (-6.6675, 168.5925) -> (-6.0325, 168.5925)
  line L493 (-6.0325, 168.5925) -> (-6.0325, 169.2275)
  line L494 (-6.6675, 169.2275) -> (-6.6675, 168.5925)
  line L495 (-6.0325, 169.2275) -> (-6.6675, 169.2275)
  line L496 (-6.0325, 169.2275) -> (-6.6675, 168.5925) construction
  line L497 (-6.6675, 169.2275) -> (-6.0325, 168.5925) construction
  line L498 (-4.1275, 168.5925) -> (-3.4925, 168.5925)
  line L499 (-3.4925, 168.5925) -> (-3.4925, 169.2275)
  line L500 (-4.1275, 169.2275) -> (-4.1275, 168.5925)
  line L501 (-3.4925, 169.2275) -> (-4.1275, 169.2275)
  line L502 (-3.4925, 169.2275) -> (-4.1275, 168.5925) construction
  line L503 (-4.1275, 169.2275) -> (-3.4925, 168.5925) construction
  line L504 (-1.5875, 168.5925) -> (-0.9525, 168.5925)
  line L505 (-0.9525, 168.5925) -> (-0.9525, 169.2275)
  line L506 (-1.5875, 169.2275) -> (-1.5875, 168.5925)
  line L507 (-0.9525, 169.2275) -> (-1.5875, 169.2275)
  line L508 (-0.9525, 169.2275) -> (-1.5875, 168.5925) construction
  line L509 (-1.5875, 169.2275) -> (-0.9525, 168.5925) construction
  line L510 (0.9525, 168.5925) -> (1.5875, 168.5925)
  line L511 (1.5875, 168.5925) -> (1.5875, 169.2275)
  line L512 (0.9525, 169.2275) -> (0.9525, 168.5925)
  line L513 (1.5875, 169.2275) -> (0.9525, 169.2275)
  line L514 (1.5875, 169.2275) -> (0.9525, 168.5925) construction
  line L515 (0.9525, 169.2275) -> (1.5875, 168.5925) construction
  line L516 (3.4925, 168.5925) -> (4.1275, 168.5925)
  line L517 (4.1275, 168.5925) -> (4.1275, 169.2275)
  line L518 (3.4925, 169.2275) -> (3.4925, 168.5925)
  line L519 (4.1275, 169.2275) -> (3.4925, 169.2275)
  line L520 (4.1275, 169.2275) -> (3.4925, 168.5925) construction
  line L521 (3.4925, 169.2275) -> (4.1275, 168.5925) construction
  line L522 (6.0325, 168.5925) -> (6.6675, 168.5925)
  line L523 (6.6675, 168.5925) -> (6.6675, 169.2275)
  line L524 (6.0325, 169.2275) -> (6.0325, 168.5925)
  line L525 (6.6675, 169.2275) -> (6.0325, 169.2275)
  line L526 (6.6675, 169.2275) -> (6.0325, 168.5925) construction
  line L527 (6.0325, 169.2275) -> (6.6675, 168.5925) construction
  line L528 (8.5725, 168.5925) -> (9.2075, 168.5925)
  line L529 (9.2075, 168.5925) -> (9.2075, 169.2275)
  line L530 (8.5725, 169.2275) -> (8.5725, 168.5925)
  line L531 (9.2075, 169.2275) -> (8.5725, 169.2275)
  line L532 (9.2075, 169.2275) -> (8.5725, 168.5925) construction
  line L533 (8.5725, 169.2275) -> (9.2075, 168.5925) construction
  line L534 (11.1125, 168.5925) -> (11.7475, 168.5925)
  line L535 (11.7475, 168.5925) -> (11.7475, 169.2275)
  line L536 (11.1125, 169.2275) -> (11.1125, 168.5925)
  line L537 (11.7475, 169.2275) -> (11.1125, 169.2275)
  line L538 (11.7475, 169.2275) -> (11.1125, 168.5925) construction
  line L539 (11.1125, 169.2275) -> (11.7475, 168.5925) construction
  line L540 (13.6525, 168.5925) -> (14.2875, 168.5925)
  line L541 (14.2875, 168.5925) -> (14.2875, 169.2275)
  line L542 (13.6525, 169.2275) -> (13.6525, 168.5925)
  line L543 (14.2875, 169.2275) -> (13.6525, 169.2275)
  line L544 (14.2875, 169.2275) -> (13.6525, 168.5925) construction
  line L545 (13.6525, 169.2275) -> (14.2875, 168.5925) construction
  line L546 (16.1925, 168.5925) -> (16.8275, 168.5925)
  line L547 (16.8275, 168.5925) -> (16.8275, 169.2275)
  line L548 (16.1925, 169.2275) -> (16.1925, 168.5925)
  line L549 (16.8275, 169.2275) -> (16.1925, 169.2275)
  line L550 (16.8275, 169.2275) -> (16.1925, 168.5925) construction
  line L551 (16.1925, 169.2275) -> (16.8275, 168.5925) construction
  line L552 (18.7325, 168.5925) -> (19.3675, 168.5925)
  line L553 (19.3675, 168.5925) -> (19.3675, 169.2275)
  line L554 (18.7325, 169.2275) -> (18.7325, 168.5925)
  line L555 (19.3675, 169.2275) -> (18.7325, 169.2275)
  line L556 (19.3675, 169.2275) -> (18.7325, 168.5925) construction
  line L557 (18.7325, 169.2275) -> (19.3675, 168.5925) construction
  line L558 (21.2725, 168.5925) -> (21.9075, 168.5925)
  line L559 (21.9075, 168.5925) -> (21.9075, 169.2275)
  line L560 (21.2725, 169.2275) -> (21.2725, 168.5925)
  line L561 (21.9075, 169.2275) -> (21.2725, 169.2275)
  line L562 (21.9075, 169.2275) -> (21.2725, 168.5925) construction
  line L563 (21.2725, 169.2275) -> (21.9075, 168.5925) construction
  line L564 (23.8125, 168.5925) -> (24.4475, 168.5925)
  line L565 (24.4475, 168.5925) -> (24.4475, 169.2275)
  line L566 (23.8125, 169.2275) -> (23.8125, 168.5925)
  line L567 (24.4475, 169.2275) -> (23.8125, 169.2275)
  line L568 (24.4475, 169.2275) -> (23.8125, 168.5925) construction
  line L569 (23.8125, 169.2275) -> (24.4475, 168.5925) construction
  line L570 (26.3525, 168.5925) -> (26.9875, 168.5925)
  line L571 (26.9875, 168.5925) -> (26.9875, 169.2275)
  line L572 (26.3525, 169.2275) -> (26.3525, 168.5925)
  line L573 (26.9875, 169.2275) -> (26.3525, 169.2275)
  line L574 (26.9875, 169.2275) -> (26.3525, 168.5925) construction
  line L575 (26.3525, 169.2275) -> (26.9875, 168.5925) construction
  line L576 (28.8925, 168.5925) -> (29.5275, 168.5925)
  line L577 (29.5275, 168.5925) -> (29.5275, 169.2275)
  line L578 (28.8925, 169.2275) -> (28.8925, 168.5925)
  line L579 (29.5275, 169.2275) -> (28.8925, 169.2275)
  line L580 (29.5275, 169.2275) -> (28.8925, 168.5925) construction
  line L581 (28.8925, 169.2275) -> (29.5275, 168.5925) construction
  line L582 (31.4325, 168.5925) -> (32.0675, 168.5925)
  line L583 (32.0675, 168.5925) -> (32.0675, 169.2275)
  line L584 (31.4325, 169.2275) -> (31.4325, 168.5925)
  line L585 (32.0675, 169.2275) -> (31.4325, 169.2275)
  line L586 (32.0675, 169.2275) -> (31.4325, 168.5925) construction
  line L587 (31.4325, 169.2275) -> (32.0675, 168.5925) construction
  line L588 (33.9725, 168.5925) -> (34.6075, 168.5925)
  line L589 (34.6075, 168.5925) -> (34.6075, 169.2275)
  line L590 (33.9725, 169.2275) -> (33.9725, 168.5925)
  line L591 (34.6075, 169.2275) -> (33.9725, 169.2275)
  line L592 (34.6075, 169.2275) -> (33.9725, 168.5925) construction
  line L593 (33.9725, 169.2275) -> (34.6075, 168.5925) construction
  line L594 (36.5125, 168.5925) -> (37.1475, 168.5925)
  line L595 (37.1475, 168.5925) -> (37.1475, 169.2275)
  line L596 (36.5125, 169.2275) -> (36.5125, 168.5925)
  line L597 (37.1475, 169.2275) -> (36.5125, 169.2275)
  line L598 (37.1475, 169.2275) -> (36.5125, 168.5925) construction
  line L599 (36.5125, 169.2275) -> (37.1475, 168.5925) construction
  line L600 (39.0525, 168.5925) -> (39.6875, 168.5925)
  line L601 (39.6875, 168.5925) -> (39.6875, 169.2275)
  line L602 (39.0525, 169.2275) -> (39.0525, 168.5925)
  line L603 (39.6875, 169.2275) -> (39.0525, 169.2275)
  line L604 (39.6875, 169.2275) -> (39.0525, 168.5925) construction
  line L605 (39.0525, 169.2275) -> (39.6875, 168.5925) construction
  line L606 (-39.6875, 171.1325) -> (-39.0525, 171.1325)
  line L607 (-39.0525, 171.1325) -> (-39.0525, 171.7675)
  line L608 (-39.6875, 171.7675) -> (-39.6875, 171.1325)
  line L609 (-39.0525, 171.7675) -> (-39.6875, 171.7675)
  line L610 (-39.0525, 171.7675) -> (-39.6875, 171.1325) construction
  line L611 (-39.6875, 171.7675) -> (-39.0525, 171.1325) construction
  line L612 (-37.1475, 171.1325) -> (-36.5125, 171.1325)
  line L613 (-36.5125, 171.1325) -> (-36.5125, 171.7675)
  line L614 (-37.1475, 171.7675) -> (-37.1475, 171.1325)
  line L615 (-36.5125, 171.7675) -> (-37.1475, 171.7675)
  line L616 (-36.5125, 171.7675) -> (-37.1475, 171.1325) construction
  line L617 (-37.1475, 171.7675) -> (-36.5125, 171.1325) construction
  line L618 (-34.6075, 171.1325) -> (-33.9725, 171.1325)
  line L619 (-33.9725, 171.1325) -> (-33.9725, 171.7675)
  line L620 (-34.6075, 171.7675) -> (-34.6075, 171.1325)
  line L621 (-33.9725, 171.7675) -> (-34.6075, 171.7675)
  line L622 (-33.9725, 171.7675) -> (-34.6075, 171.1325) construction
  line L623 (-34.6075, 171.7675) -> (-33.9725, 171.1325) construction
  line L624 (-32.0675, 171.1325) -> (-31.4325, 171.1325)
  line L625 (-31.4325, 171.1325) -> (-31.4325, 171.7675)
  line L626 (-32.0675, 171.7675) -> (-32.0675, 171.1325)
  line L627 (-31.4325, 171.7675) -> (-32.0675, 171.7675)
  line L628 (-31.4325, 171.7675) -> (-32.0675, 171.1325) construction
  line L629 (-32.0675, 171.7675) -> (-31.4325, 171.1325) construction
  line L630 (-29.5275, 171.1325) -> (-28.8925, 171.1325)
  line L631 (-28.8925, 171.1325) -> (-28.8925, 171.7675)
  line L632 (-29.5275, 171.7675) -> (-29.5275, 171.1325)
  line L633 (-28.8925, 171.7675) -> (-29.5275, 171.7675)
  line L634 (-28.8925, 171.7675) -> (-29.5275, 171.1325) construction
  line L635 (-29.5275, 171.7675) -> (-28.8925, 171.1325) construction
  line L636 (-26.9875, 171.1325) -> (-26.3525, 171.1325)
  line L637 (-26.3525, 171.1325) -> (-26.3525, 171.7675)
  line L638 (-26.9875, 171.7675) -> (-26.9875, 171.1325)
  line L639 (-26.3525, 171.7675) -> (-26.9875, 171.7675)
  line L640 (-26.3525, 171.7675) -> (-26.9875, 171.1325) construction
  line L641 (-26.9875, 171.7675) -> (-26.3525, 171.1325) construction
  line L642 (-24.4475, 171.1325) -> (-23.8125, 171.1325)
  line L643 (-23.8125, 171.1325) -> (-23.8125, 171.7675)
  line L644 (-24.4475, 171.7675) -> (-24.4475, 171.1325)
  line L645 (-23.8125, 171.7675) -> (-24.4475, 171.7675)
  line L646 (-23.8125, 171.7675) -> (-24.4475, 171.1325) construction
  line L647 (-24.4475, 171.7675) -> (-23.8125, 171.1325) construction
  line L648 (-21.9075, 171.1325) -> (-21.2725, 171.1325)
  line L649 (-21.2725, 171.1325) -> (-21.2725, 171.7675)
  line L650 (-21.9075, 171.7675) -> (-21.9075, 171.1325)
  line L651 (-21.2725, 171.7675) -> (-21.9075, 171.7675)
  line L652 (-21.2725, 171.7675) -> (-21.9075, 171.1325) construction
  line L653 (-21.9075, 171.7675) -> (-21.2725, 171.1325) construction
  line L654 (-19.3675, 171.1325) -> (-18.7325, 171.1325)
  line L655 (-18.7325, 171.1325) -> (-18.7325, 171.7675)
  line L656 (-19.3675, 171.7675) -> (-19.3675, 171.1325)
  line L657 (-18.7325, 171.7675) -> (-19.3675, 171.7675)
  line L658 (-18.7325, 171.7675) -> (-19.3675, 171.1325) construction
  line L659 (-19.3675, 171.7675) -> (-18.7325, 171.1325) construction
  line L660 (-16.8275, 171.1325) -> (-16.1925, 171.1325)
  line L661 (-16.1925, 171.1325) -> (-16.1925, 171.7675)
  line L662 (-16.8275, 171.7675) -> (-16.8275, 171.1325)
  line L663 (-16.1925, 171.7675) -> (-16.8275, 171.7675)
  line L664 (-16.1925, 171.7675) -> (-16.8275, 171.1325) construction
  line L665 (-16.8275, 171.7675) -> (-16.1925, 171.1325) construction
  line L666 (-14.2875, 171.1325) -> (-13.6525, 171.1325)
  line L667 (-13.6525, 171.1325) -> (-13.6525, 171.7675)
  line L668 (-14.2875, 171.7675) -> (-14.2875, 171.1325)
  line L669 (-13.6525, 171.7675) -> (-14.2875, 171.7675)
  line L670 (-13.6525, 171.7675) -> (-14.2875, 171.1325) construction
  line L671 (-14.2875, 171.7675) -> (-13.6525, 171.1325) construction
  line L672 (-11.7475, 171.1325) -> (-11.1125, 171.1325)
  line L673 (-11.1125, 171.1325) -> (-11.1125, 171.7675)
  line L674 (-11.7475, 171.7675) -> (-11.7475, 171.1325)
  line L675 (-11.1125, 171.7675) -> (-11.7475, 171.7675)
  line L676 (-11.1125, 171.7675) -> (-11.7475, 171.1325) construction
  line L677 (-11.7475, 171.7675) -> (-11.1125, 171.1325) construction
  line L678 (-9.2075, 171.1325) -> (-8.5725, 171.1325)
  line L679 (-8.5725, 171.1325) -> (-8.5725, 171.7675)
  line L680 (-9.2075, 171.7675) -> (-9.2075, 171.1325)
  line L681 (-8.5725, 171.7675) -> (-9.2075, 171.7675)
  line L682 (-8.5725, 171.7675) -> (-9.2075, 171.1325) construction
  line L683 (-9.2075, 171.7675) -> (-8.5725, 171.1325) construction
  line L684 (-6.6675, 171.1325) -> (-6.0325, 171.1325)
  line L685 (-6.0325, 171.1325) -> (-6.0325, 171.7675)
  line L686 (-6.6675, 171.7675) -> (-6.6675, 171.1325)
  line L687 (-6.0325, 171.7675) -> (-6.6675, 171.7675)
  line L688 (-6.0325, 171.7675) -> (-6.6675, 171.1325) construction
  line L689 (-6.6675, 171.7675) -> (-6.0325, 171.1325) construction
  line L690 (-4.1275, 171.1325) -> (-3.4925, 171.1325)
  line L691 (-3.4925, 171.1325) -> (-3.4925, 171.7675)
  line L692 (-4.1275, 171.7675) -> (-4.1275, 171.1325)
  line L693 (-3.4925, 171.7675) -> (-4.1275, 171.7675)
  line L694 (-3.4925, 171.7675) -> (-4.1275, 171.1325) construction
  line L695 (-4.1275, 171.7675) -> (-3.4925, 171.1325) construction
  line L696 (-1.5875, 171.1325) -> (-0.9525, 171.1325)
  line L697 (-0.9525, 171.1325) -> (-0.9525, 171.7675)
  line L698 (-1.5875, 171.7675) -> (-1.5875, 171.1325)
  line L699 (-0.9525, 171.7675) -> (-1.5875, 171.7675)
  line L700 (-0.9525, 171.7675) -> (-1.5875, 171.1325) construction
  line L701 (-1.5875, 171.7675) -> (-0.9525, 171.1325) construction
  line L702 (0.9525, 171.1325) -> (1.5875, 171.1325)
  line L703 (1.5875, 171.1325) -> (1.5875, 171.7675)
  line L704 (0.9525, 171.7675) -> (0.9525, 171.1325)
  line L705 (1.5875, 171.7675) -> (0.9525, 171.7675)
  line L706 (1.5875, 171.7675) -> (0.9525, 171.1325) construction
  line L707 (0.9525, 171.7675) -> (1.5875, 171.1325) construction
  line L708 (3.4925, 171.1325) -> (4.1275, 171.1325)
  line L709 (4.1275, 171.1325) -> (4.1275, 171.7675)
  line L710 (3.4925, 171.7675) -> (3.4925, 171.1325)
  line L711 (4.1275, 171.7675) -> (3.4925, 171.7675)
  line L712 (4.1275, 171.7675) -> (3.4925, 171.1325) construction
  line L713 (3.4925, 171.7675) -> (4.1275, 171.1325) construction
  line L714 (6.0325, 171.1325) -> (6.6675, 171.1325)
  line L715 (6.6675, 171.1325) -> (6.6675, 171.7675)
  line L716 (6.0325, 171.7675) -> (6.0325, 171.1325)
  line L717 (6.6675, 171.7675) -> (6.0325, 171.7675)
  line L718 (6.6675, 171.7675) -> (6.0325, 171.1325) construction
  line L719 (6.0325, 171.7675) -> (6.6675, 171.1325) construction
  line L720 (8.5725, 171.1325) -> (9.2075, 171.1325)
  line L721 (9.2075, 171.1325) -> (9.2075, 171.7675)
  line L722 (8.5725, 171.7675) -> (8.5725, 171.1325)
  line L723 (9.2075, 171.7675) -> (8.5725, 171.7675)
  line L724 (9.2075, 171.7675) -> (8.5725, 171.1325) construction
  line L725 (8.5725, 171.7675) -> (9.2075, 171.1325) construction
  line L726 (11.1125, 171.1325) -> (11.7475, 171.1325)
  line L727 (11.7475, 171.1325) -> (11.7475, 171.7675)
  line L728 (11.1125, 171.7675) -> (11.1125, 171.1325)
  line L729 (11.7475, 171.7675) -> (11.1125, 171.7675)
  line L730 (11.7475, 171.7675) -> (11.1125, 171.1325) construction
  line L731 (11.1125, 171.7675) -> (11.7475, 171.1325) construction
  line L732 (13.6525, 171.1325) -> (14.2875, 171.1325)
  line L733 (14.2875, 171.1325) -> (14.2875, 171.7675)
  line L734 (13.6525, 171.7675) -> (13.6525, 171.1325)
  line L735 (14.2875, 171.7675) -> (13.6525, 171.7675)
  line L736 (14.2875, 171.7675) -> (13.6525, 171.1325) construction
  line L737 (13.6525, 171.7675) -> (14.2875, 171.1325) construction
  line L738 (16.1925, 171.1325) -> (16.8275, 171.1325)
  line L739 (16.8275, 171.1325) -> (16.8275, 171.7675)
  line L740 (16.1925, 171.7675) -> (16.1925, 171.1325)
  line L741 (16.8275, 171.7675) -> (16.1925, 171.7675)
  line L742 (16.8275, 171.7675) -> (16.1925, 171.1325) construction
  line L743 (16.1925, 171.7675) -> (16.8275, 171.1325) construction
  line L744 (18.7325, 171.1325) -> (19.3675, 171.1325)
  line L745 (19.3675, 171.1325) -> (19.3675, 171.7675)
  line L746 (18.7325, 171.7675) -> (18.7325, 171.1325)
  line L747 (19.3675, 171.7675) -> (18.7325, 171.7675)
  line L748 (19.3675, 171.7675) -> (18.7325, 171.1325) construction
  line L749 (18.7325, 171.7675) -> (19.3675, 171.1325) construction
  line L750 (21.2725, 171.1325) -> (21.9075, 171.1325)
  line L751 (21.9075, 171.1325) -> (21.9075, 171.7675)
  line L752 (21.2725, 171.7675) -> (21.2725, 171.1325)
  line L753 (21.9075, 171.7675) -> (21.2725, 171.7675)
  line L754 (21.9075, 171.7675) -> (21.2725, 171.1325) construction
  line L755 (21.2725, 171.7675) -> (21.9075, 171.1325) construction